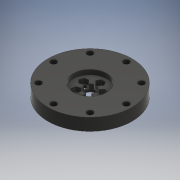
# Autodesk Inventor part: XT-SM-02
Saved by Autodesk Inventor 2017 (Build 210142000, 142)
## iProperties
Created: 2019-11-11
Part Number: XT-SM-02
Material: ABS Plastic
Document SubType Name: Modeling
Designer: Dell
Density: 1.06 g/cm^3
Appearance: Smooth - Black
Author: Dell
Autodesk Inventor part; units mm, degrees
ref_plane "YZ Plane" through (0, 0, 0) normal (1, 0, 0) x (0, 1, 0)
ref_plane "XZ Plane" through (0, 0, 0) normal (0, 1, 0) x (-1, 0, 0)
ref_plane "XY Plane" through (0, 0, 0) normal (0, 0, 1) x (1, 0, 0)
sketch "Sketch1" plane through (0, 0, 0) normal (0, 0, 1) x (1, 0, 0)
  circle A0 centre (0, 0) radius 34.05
  circle A1 centre (0, 0) radius 5
  circle A2 centre (29.5, 0) radius 2.5
  circle A3 centre (20.8597, 20.8597) radius 2.5
  circle A4 centre (0, 29.5) radius 2.5
  circle A5 centre (-20.8597, 20.8597) radius 2.5
  circle A6 centre (-29.5, 0) radius 2.5
  circle A7 centre (-20.8597, -20.8597) radius 2.5
  circle A8 centre (0, -29.5) radius 2.5
  circle A9 centre (20.8597, -20.8597) radius 2.5
  circle A10 centre (0, 8) radius 2
  circle A11 centre (-7.6085, 2.4721) radius 2
  circle A12 centre (-4.7023, -6.4721) radius 2
  circle A13 centre (4.7023, -6.4721) radius 2
  circle A14 centre (7.6085, 2.4721) radius 2
  dimension "d0" = 68.1
  dimension "d1" = 10
  dimension "d2" = 5
  dimension "d3" = 29.5
  dimension "d6" = 360
  dimension "d8" = 4
  dimension "d9" = 8
  dimension "d12" = 360
  constraints: 15 centre point, 2 coincident, 1 horizontal alignment, 1 vertical alignment, 28 other
  measures "d0" diameter of A0
  measures "d1" diameter of A1
  measures "d2" diameter of A2
  measures "d3" distance of A2.centre point (0, 0)
  measures "d8" diameter of A10
  measures "d9" distance of A10.centre point (0, 0)
extrude "Extrusion1" add sketch "Sketch1" along normal blind 10
sketch "Sketch2" plane through (0, 0, 10) normal (0, 0, 1) x (1, 0, 0)
  line L0 (-3.4641, 8) -> (-1.7321, 11)
  line L1 (-1.7321, 11) -> (1.7321, 11)
  line L2 (1.7321, 11) -> (3.4641, 8)
  line L3 (3.4641, 8) -> (1.7321, 5)
  line L4 (1.7321, 5) -> (-1.7321, 5)
  line L5 (-1.7321, 5) -> (-3.4641, 8)
  circle A0 centre (0, 8) radius 2 projected
  line L6 (-8.6789, -0.8224) -> (-10.9969, 1.7519)
  line L7 (-10.9969, 1.7519) -> (-9.9264, 5.0465)
  line L8 (-9.9264, 5.0465) -> (-6.538, 5.7667)
  line L9 (-6.538, 5.7667) -> (-4.22, 3.1924)
  line L10 (-4.22, 3.1924) -> (-5.2905, -0.1022)
  line L11 (-5.2905, -0.1022) -> (-8.6789, -0.8224)
  line L12 (-1.8998, -8.5083) -> (-5.0644, -9.9173)
  line L13 (-5.0644, -9.9173) -> (-7.8669, -7.8811)
  line L14 (-7.8669, -7.8811) -> (-7.5048, -4.436)
  line L15 (-7.5048, -4.436) -> (-4.3402, -3.027)
  line L16 (-4.3402, -3.027) -> (-1.5377, -5.0632)
  line L17 (-1.5377, -5.0632) -> (-1.8998, -8.5083)
  line L18 (7.5048, -4.436) -> (7.8669, -7.8811)
  line L19 (7.8669, -7.8811) -> (5.0644, -9.9173)
  line L20 (5.0644, -9.9173) -> (1.8998, -8.5083)
  line L21 (1.8998, -8.5083) -> (1.5377, -5.0632)
  line L22 (1.5377, -5.0632) -> (4.3402, -3.027)
  line L23 (4.3402, -3.027) -> (7.5048, -4.436)
  line L24 (6.538, 5.7667) -> (9.9264, 5.0465)
  line L25 (9.9264, 5.0465) -> (10.9969, 1.7519)
  line L26 (10.9969, 1.7519) -> (8.6789, -0.8224)
  line L27 (8.6789, -0.8224) -> (5.2905, -0.1022)
  line L28 (5.2905, -0.1022) -> (4.22, 3.1924)
  line L29 (4.22, 3.1924) -> (6.538, 5.7667)
  point P0 (0, 0)
  point P1 (-7.6085, 2.4721)
  point P2 (-4.7023, -6.4721)
  point P3 (4.7023, -6.4721)
  point P4 (7.6085, 2.4721)
  dimension "d16" = 6
  dimension "d19" = 360
  constraints: 60 end point, 1 coincident, 1 horizontal, 79 other
  measures "d16" distance between parallel lines of L4 L1
extrude "Extrusion2" cut sketch "Sketch2" against normal blind 8 contours L0 L1 L2 L3 L4 L5 | A0 | L6 L7 L8 L9 L10 L11 | L12 L13 L14 L15 L16 L17 | L18 L19 L20 L21 L22 L23 | L24 L25 L26 L27 L28 L29
sketch "Sketch3" plane through (0, 0, 10) normal (0, 0, 1) x (1, 0, 0)
  line L0 (-1.7321, 5) -> (-3.4641, 8) projected
  line L1 (-3.4641, 8) -> (0, 2)
  line L2 (3.4641, 8) -> (1.7321, 5) projected
  line L3 (0, 2) -> (3.4641, 8)
  line L4 (1.7321, 11) -> (3.4641, 8) projected
  line L5 (-3.4641, 8) -> (3.4641, 8)
  line L6 (-8.6789, -0.8224) -> (-1.9021, 0.618)
  line L7 (-1.9021, 0.618) -> (-6.538, 5.7667)
  line L8 (-8.6789, -0.8224) -> (-6.538, 5.7667)
  line L9 (-1.8998, -8.5083) -> (-1.1756, -1.618)
  line L10 (-1.1756, -1.618) -> (-7.5048, -4.436)
  line L11 (-1.8998, -8.5083) -> (-7.5048, -4.436)
  line L12 (7.5048, -4.436) -> (1.1756, -1.618)
  line L13 (1.1756, -1.618) -> (1.8998, -8.5083)
  line L14 (7.5048, -4.436) -> (1.8998, -8.5083)
  line L15 (6.538, 5.7667) -> (1.9021, 0.618)
  line L16 (1.9021, 0.618) -> (8.6789, -0.8224)
  line L17 (6.538, 5.7667) -> (8.6789, -0.8224)
  point P0 (0, 0)
  point P1 (-4.22, 3.1924)
  point P2 (-4.3402, -3.027)
  point P3 (1.5377, -5.0632)
  point P4 (5.2905, -0.1022)
  dimension "d25" = 360
  constraints: 30 end point, 5 midpoint, 1 collinear, 1 horizontal, 36 other
extrude "Extrusion3" cut sketch "Sketch3" against normal up to surface (8 mm away) from surface at 0
sketch "Sketch4" plane through (0, 0, 10) normal (0, 0, 1) x (1, 0, 0)
  circle A0 centre (0, 0) radius 13.5
  dimension "d29" = 27
  constraints: 1 centre point, 1 coincident
  measures "d29" diameter of A0
extrude "Extrusion4" cut sketch "Sketch4" against normal blind 4
body "Solid1"
